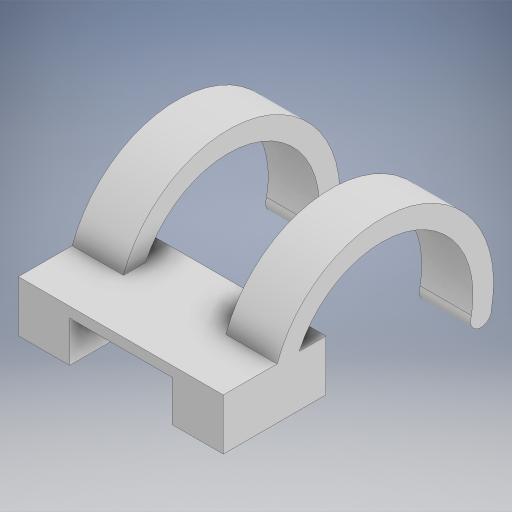
# Autodesk Inventor part: Hook
Saved by Autodesk Inventor 2024.2 (Build 282272000, 272)
## iProperties
Created: 2024-03-09
Part Number: Hook
Material: Generic
Document SubType Name: Modeling
Designer: rohan
Density: 1 g/cm^3
Appearance: Default
Author: rohan
Autodesk Inventor part; units mm, degrees
ref_plane "YZ Plane" through (0, 0, 0) normal (1, 0, 0) x (0, 1, 0)
ref_plane "XZ Plane" through (0, 0, 0) normal (0, 1, 0) x (-1, 0, 0)
ref_plane "XY Plane" through (0, 0, 0) normal (0, 0, 1) x (1, 0, 0)
sketch "Sketch2" plane through (0, 0, 0) normal (1, 0, 0) x (0, 1, 0)
  line L0 (4.8096, 10.1352) -> (-7.8904, 10.1352)
  line L1 (-7.8904, 10.1352) -> (-7.8904, -15.2648)
  line L2 (-7.8904, -15.2648) -> (4.8096, -15.2648)
  line L3 (4.8096, -15.2648) -> (4.8096, 10.1352)
  arc A0 (-8.905, -51.3869) -> (4.8096, -8.6933) centre (-4.5952, -29.2218) ccw
  arc A1 (-9.8746, -56.3735) -> (4.8096, -3.2095) centre (-4.5952, -29.2218) ccw
  arc A2 (-8.905, -51.3869) -> (-9.8746, -56.3735) centre (-10.049, -53.7521) ccw
  point P0 (0, 0)
  dimension "d4" = 12.7
  dimension "d5" = 25.4
  dimension "d6" = 5.08
  constraints: 8 end point, 6 point on circle, 3 centre point, 2 parallel, 2 point on line, 1 horizontal, 1 perpendicular
  measures "d4" distance of L2.end L1.end
  measures "d5" distance of L1.end L0.end
  measures "d6" radial gap between concentric circles of A0 A1
extrude "Extrusion2" add sketch "Sketch2" along normal blind 12.7
ref_plane "Work Plane1" through (25.4, 0, 0) normal (1, 0, 0) x (0, 0, -1)
mirror "Mirror1" about plane through (25.4, 0, 0) normal (1, 0, 0) of "Extrusion2"
sketch "Sketch3" plane through (12.7, 0, 0) normal (1, 0, 0) x (0, 0, -1)
  line L0 (3.2095, 4.8096) -> (-10.1352, 4.8096) projected
  line L1 (15.2648, -7.8904) -> (15.2648, 4.8096) projected
  line L2 (-10.1352, 4.8096) -> (15.2648, 4.8096)
  line L3 (15.2648, 4.8096) -> (15.2648, 2.2696)
  line L4 (15.2648, 2.2696) -> (-10.1352, 2.2696)
  line L5 (-10.1352, 2.2696) -> (-10.1352, 4.8096)
  point P0 (0, 0)
  point P1 (15.2648, 4.8096)
  dimension "d10" = 2.54
  constraints: 8 end point, 2 parallel, 1 horizontal, 1 perpendicular, 1 point on line
  measures "d10" distance between parallel lines of L0 L4
extrude "Extrusion3" add sketch "Sketch3" along normal up to surface (25.4 mm away)
body "Solid2"
